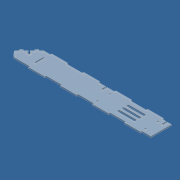
# Autodesk Inventor part: Wall
Saved by Autodesk Inventor 2016 (Build 200138000, 138)
## iProperties
Created: 2016-04-03
Part Number: Wall
Material: Polycarbonate, Clear
Document SubType Name: Modeling
Designer: admin
Density: 1.2 g/cm^3
Appearance: Polycarbonate - Clear
Author: admin
Autodesk Inventor part; units mm, degrees
ref_plane "YZ Plane" through (0, 0, 0) normal (1, 0, 0) x (0, 1, 0)
ref_plane "XZ Plane" through (0, 0, 0) normal (0, 1, 0) x (-1, 0, 0)
ref_plane "XY Plane" through (0, 0, 0) normal (0, 0, 1) x (1, 0, 0)
sketch "Sketch1" plane through (0, 0, 0) normal (0, 0, 1) x (1, 0, 0)
  line L0 (142.5, -22.5) -> (142.5, 22.5)
  arc A0 (-169.3198, -9.3198) -> (-157.5, -22.5) centre (-130.5627, 13.547) ccw
  line L1 (-154.4706, 5.5294) -> (-150.935, 1.9939)
  line L2 (-150.935, 1.9939) -> (-152.2157, 0.7132)
  line L3 (-152.2157, 0.7132) -> (-150.8015, -0.701)
  line L4 (-150.8015, -0.701) -> (-149.5208, 0.5797)
  line L5 (-149.5208, 0.5797) -> (-147.3995, -1.5416)
  line L6 (-147.3995, -1.5416) -> (-145.2782, 0.5797)
  line L7 (-145.2782, 0.5797) -> (-147.3995, 2.701)
  line L8 (-147.3995, 2.701) -> (-146.1188, 3.9817)
  line L9 (-146.1188, 3.9817) -> (-147.533, 5.3959)
  line L10 (-147.533, 5.3959) -> (-148.8137, 4.1152)
  line L11 (-148.8137, 4.1152) -> (-152.3492, 7.6508)
  line L12 (-154.542, 7.7222) -> (-156.666, 9.8462) construction
  line L13 (-122.5, 22.5) -> (-122.5, 25.5)
  line L14 (-122.5, 25.5) -> (-87.5, 25.5)
  line L15 (-87.5, 25.5) -> (-87.5, 22.5)
  line L16 (-52.5, 22.5) -> (-52.5, 25.5)
  line L17 (-52.5, 25.5) -> (-17.5, 25.5)
  line L18 (-17.5, 25.5) -> (-17.5, 22.5)
  line L19 (17.5, 22.5) -> (17.5, 25.5)
  line L20 (17.5, 25.5) -> (52.5, 25.5)
  line L21 (52.5, 25.5) -> (52.5, 22.5)
  line L22 (87.5, 22.5) -> (87.5, 25.5)
  line L23 (87.5, 25.5) -> (122.5, 25.5)
  line L24 (122.5, 25.5) -> (122.5, 22.5)
  line L25 (87.5, 22.5) -> (52.5, 22.5)
  line L26 (-52.5, 22.5) -> (-87.5, 22.5)
  line L27 (-122.5, 22.5) -> (-137.5, 22.5)
  line L28 (-122.5, -22.5) -> (-122.5, -25.5)
  line L29 (-122.5, -25.5) -> (-87.5, -25.5)
  line L30 (-87.5, -25.5) -> (-87.5, -22.5)
  line L31 (-52.5, -22.5) -> (-52.5, -25.5)
  line L32 (-52.5, -25.5) -> (-17.5, -25.5)
  line L33 (-17.5, -25.5) -> (-17.5, -22.5)
  line L34 (17.5, -22.5) -> (17.5, -25.5)
  line L35 (17.5, -25.5) -> (52.5, -25.5)
  line L36 (52.5, -25.5) -> (52.5, -22.5)
  line L37 (87.5, -22.5) -> (87.5, -25.5)
  line L38 (87.5, -25.5) -> (122.5, -25.5)
  line L39 (122.5, -25.5) -> (122.5, -22.5)
  line L40 (-157.5, -22.5) -> (-122.5, -22.5)
  line L41 (-87.5, -22.5) -> (-52.5, -22.5)
  line L42 (-17.5, -22.5) -> (17.5, -22.5)
  line L43 (52.5, -22.5) -> (87.5, -22.5)
  line L44 (122.5, -22.5) -> (142.5, -22.5)
  line L45 (-1.5, 12.5) -> (-1.5, 22.5)
  line L46 (1.5, 22.5) -> (1.5, 12.5)
  line L47 (1.5, 12.5) -> (-1.5, 12.5)
  line L48 (-37.337, 0) -> (-30.889, 0) construction
  line L49 (-164.0165, -4.0165) -> (-166.1378, -1.8952)
  line L50 (-166.1378, -1.8952) -> (-161.8952, 2.3475)
  line L51 (-161.8952, 2.3475) -> (-159.7739, 0.2261)
  line L52 (-147.0459, 12.9541) -> (-149.1673, 15.0754)
  line L53 (-149.1673, 15.0754) -> (-144.9246, 19.318)
  line L54 (-144.9246, 19.318) -> (-142.8033, 17.1967)
  line L55 (-154.4706, 5.5294) -> (-159.7739, 0.2261)
  line L56 (-164.0165, -4.0165) -> (-169.3198, -9.3198)
  line L57 (-137.5, 22.5) -> (-142.8033, 17.1967)
  line L58 (-147.0459, 12.9541) -> (-152.3492, 7.6508)
  line L59 (17.5, 22.5) -> (1.5, 22.5)
  line L60 (-1.5, 22.5) -> (-17.5, 22.5)
  line L61 (131, 22.5) -> (131, 12.5)
  line L62 (131, 12.5) -> (134, 12.5)
  line L63 (134, 12.5) -> (134, 22.5)
  line L64 (122.5, 22.5) -> (131, 22.5)
  line L65 (134, 22.5) -> (142.5, 22.5)
  point P0 (0, 0)
  point P1 (142.5, 0)
  point P2 (-146.3388, -0.481)
  point P3 (0, -22.5)
  point P4 (1.5, -22.5)
  dimension "d0" = 45
  dimension "d2" = 45
  dimension "d4" = 45
  dimension "d7" = 3
  dimension "d8" = 2
  dimension "d9" = 3
  dimension "d10" = 5
  dimension "d11" = 6.6223
  dimension "d13" = 35
  dimension "d15" = 20
  dimension "d17" = 10
  dimension "d23" = 45
  dimension "d24" = 6
  dimension "d25" = 18
  dimension "d35" = 3
  dimension "d36" = 35
  dimension "d37" = 15
  dimension "d38" = 300
  dimension "d40" = 8.5
  constraints: 132 end point, 72 perpendicular, 33 collinear, 16 equal length, 8 horizontal, 6 parallel, 5 vertical, 3 midpoint, 2 point on circle, 2 point on line, 1 centre point, 1 horizontal alignment, 1 vertical alignment, 2 other
  measures "d0" distance of L0.start L0.end
  measures "d2" distance of L56.end L27.end
  measures "d4" radius of A0
  measures "d7" distance between parallel lines of L7 L5
  measures "d8" distance between parallel lines of L8 L10
  measures "d9" distance of L6.end L7.end
  measures "d10" distance of L10.end L11.end
  measures "d11" distance between parallel lines of L9 L3
  measures "d13" distance of L13.end L14.end
  measures "d15" distance from line of L23.end L0
  measures "d17" distance of L45.start L45.end
  measures "d23" angle of L40 L56
  measures "d24" distance of L49.end L50.end
  measures "d25" distance between parallel lines of L52 L51
  measures "d35" distance of L22.start L22.end
  measures "d36" distance of L19.start L18.end
  measures "d37" distance of L13.start L27.end
  measures "d38" distance from line of L0 L40.start
  measures "d40" distance between parallel lines of L0 L63
extrude "Extrusion1" add sketch "Sketch1" along normal blind 3
sketch "Sketch2" plane through (0, 0, 3) normal (0, 0, 1) x (1, 0, 0)
  line L0 (1.5, 22.5) -> (1.5, 12.5) projected
  line L1 (142.5, -22.5) -> (142.5, 22.5) projected
  line L2 (122.5, 22.5) -> (122.5, 25.5) projected
  line L3 (122.5, 25.5) -> (87.5, 25.5) projected
  line L4 (87.5, 25.5) -> (87.5, 22.5) projected
  line L5 (87.5, 22.5) -> (52.5, 22.5) projected
  line L6 (52.5, 22.5) -> (52.5, 25.5) projected
  line L7 (52.5, 25.5) -> (17.5, 25.5) projected
  line L8 (17.5, 25.5) -> (17.5, 22.5) projected
  line L9 (17.5, 22.5) -> (1.5, 22.5) projected
  line L10 (-17.5, -22.5) -> (17.5, -22.5) projected
  line L11 (17.5, -22.5) -> (17.5, -25.5) projected
  line L12 (17.5, -25.5) -> (52.5, -25.5) projected
  line L13 (52.5, -25.5) -> (52.5, -22.5) projected
  line L14 (52.5, -22.5) -> (87.5, -22.5) projected
  line L15 (87.5, -22.5) -> (87.5, -25.5) projected
  line L16 (87.5, -25.5) -> (122.5, -25.5) projected
  line L17 (122.5, -25.5) -> (122.5, -22.5) projected
  line L18 (122.5, -22.5) -> (142.5, -22.5) projected
  line L19 (-125.5, 10) -> (-125.5, -10)
  line L20 (131, 22.5) -> (122.5, 22.5) projected
  line L21 (1.5, 12.5) -> (-1.5, 12.5) projected
  line L22 (-1.5, 12.5) -> (-1.5, 22.5) projected
  line L23 (-1.5, 22.5) -> (-17.5, 22.5) projected
  line L24 (-17.5, 22.5) -> (-17.5, 25.5) projected
  line L25 (-17.5, 25.5) -> (-52.5, 25.5) projected
  line L26 (-52.5, 25.5) -> (-52.5, 22.5) projected
  line L27 (-52.5, 22.5) -> (-87.5, 22.5) projected
  line L28 (-87.5, 22.5) -> (-87.5, 25.5) projected
  line L29 (-87.5, 25.5) -> (-122.5, 25.5) projected
  line L30 (-122.5, 25.5) -> (-122.5, 22.5) projected
  line L31 (-122.5, -25.5) -> (-87.5, -25.5) projected
  line L32 (-87.5, -25.5) -> (-87.5, -22.5) projected
  line L33 (-87.5, -22.5) -> (-52.5, -22.5) projected
  line L34 (-52.5, -22.5) -> (-52.5, -25.5) projected
  line L35 (-52.5, -25.5) -> (-17.5, -25.5) projected
  line L36 (-17.5, -25.5) -> (-17.5, -22.5) projected
  line L37 (-122.5, 22.5) -> (-137.5, 22.5) projected
  line L38 (-137.5, 22.5) -> (-142.8033, 17.1967) projected
  line L39 (-142.8033, 17.1967) -> (-144.9246, 19.318) projected
  line L40 (-144.9246, 19.318) -> (-149.1673, 15.0754) projected
  line L41 (-149.1673, 15.0754) -> (-147.0459, 12.9541) projected
  line L42 (-147.0459, 12.9541) -> (-152.3492, 7.6508) projected
  line L43 (-152.3492, 7.6508) -> (-148.8137, 4.1152) projected
  line L44 (-148.8137, 4.1152) -> (-147.533, 5.3959) projected
  line L45 (-147.533, 5.3959) -> (-146.1188, 3.9817) projected
  line L46 (-146.1188, 3.9817) -> (-147.3995, 2.701) projected
  line L47 (-147.3995, 2.701) -> (-145.2782, 0.5797) projected
  line L48 (-157.5, -22.5) -> (-122.5, -22.5) projected
  line L49 (-122.5, -22.5) -> (-122.5, -25.5) projected
  line L50 (-145.2782, 0.5797) -> (-147.3995, -1.5416) projected
  line L51 (-147.3995, -1.5416) -> (-149.5208, 0.5797) projected
  line L52 (-149.5208, 0.5797) -> (-150.8015, -0.701) projected
  line L53 (-150.8015, -0.701) -> (-152.2157, 0.7132) projected
  line L54 (-152.2157, 0.7132) -> (-150.935, 1.9939) projected
  line L55 (-150.935, 1.9939) -> (-154.4706, 5.5294) projected
  line L56 (-154.4706, 5.5294) -> (-159.7739, 0.2261) projected
  line L57 (-159.7739, 0.2261) -> (-161.8952, 2.3475) projected
  line L58 (-161.8952, 2.3475) -> (-166.1378, -1.8952) projected
  line L59 (-166.1378, -1.8952) -> (-164.0165, -4.0165) projected
  line L60 (-164.0165, -4.0165) -> (-169.3198, -9.3198) projected
  arc A0 (-169.3198, -9.3198) -> (-157.5, -22.5) centre (-130.5627, 13.547) ccw projected
  line L61 (142.5, 22.5) -> (134, 22.5) projected
  line L62 (134, 22.5) -> (134, 12.5) projected
  line L63 (134, 12.5) -> (131, 12.5) projected
  line L64 (131, 12.5) -> (131, 22.5) projected
  line L65 (-125.5, 10) -> (-122.5, 10)
  line L66 (-122.5, 10) -> (-122.5, -10)
  line L67 (-122.5, -10) -> (-125.5, -10)
  line L68 (-87.5, 22.5) -> (-87.5, 25.5) projected
  point P0 (0, 0)
  point P1 (-125.5, 0)
  dimension "d20" = 268
  dimension "d39" = 20
  constraints: 8 end point, 2 horizontal, 1 horizontal alignment, 1 midpoint, 1 perpendicular, 1 vertical
  measures "d20" distance between parallel lines of L1 L19
  measures "d39" distance between parallel lines of L67 L65
extrude "Extrusion2" cut sketch "Sketch2" against normal blind 10 contours L65 L66 L67 L19
sketch "Sketch3" plane through (0, 0, 3) normal (0, 0, 1) x (1, 0, 0)
  line L0 (1.5, 22.5) -> (1.5, 12.5) projected
  line L1 (142.5, -22.5) -> (142.5, 22.5) projected
  line L2 (122.5, 22.5) -> (122.5, 25.5) projected
  line L3 (122.5, 25.5) -> (87.5, 25.5) projected
  line L4 (87.5, 25.5) -> (87.5, 22.5) projected
  line L5 (87.5, 22.5) -> (52.5, 22.5) projected
  line L6 (52.5, 22.5) -> (52.5, 25.5) projected
  line L7 (52.5, 25.5) -> (17.5, 25.5) projected
  line L8 (17.5, 25.5) -> (17.5, 22.5) projected
  line L9 (17.5, 22.5) -> (1.5, 22.5) projected
  line L10 (-17.5, -22.5) -> (17.5, -22.5) projected
  line L11 (17.5, -22.5) -> (17.5, -25.5) projected
  line L12 (17.5, -25.5) -> (52.5, -25.5) projected
  line L13 (52.5, -25.5) -> (52.5, -22.5) projected
  line L14 (52.5, -22.5) -> (87.5, -22.5) projected
  line L15 (87.5, -22.5) -> (87.5, -25.5) projected
  line L16 (87.5, -25.5) -> (122.5, -25.5) projected
  line L17 (122.5, -25.5) -> (122.5, -22.5) projected
  line L18 (122.5, -22.5) -> (142.5, -22.5) projected
  arc A0 (59.5166, -6.8198) -> (59.5166, -11.8198) centre (59.5166, -9.3198) ccw
  arc A1 (94.5166, -11.8198) -> (94.5166, -6.8198) centre (94.5166, -9.3198) ccw
  line L19 (59.5166, -6.8198) -> (94.5166, -6.8198)
  line L20 (59.5166, -11.8198) -> (94.5166, -11.8198)
  line L21 (131, 22.5) -> (122.5, 22.5) projected
  line L22 (1.5, 12.5) -> (-1.5, 12.5) projected
  line L23 (-1.5, 12.5) -> (-1.5, 22.5) projected
  line L24 (-1.5, 22.5) -> (-17.5, 22.5) projected
  line L25 (-17.5, 22.5) -> (-17.5, 25.5) projected
  line L26 (-17.5, 25.5) -> (-52.5, 25.5) projected
  line L27 (-52.5, 25.5) -> (-52.5, 22.5) projected
  line L28 (-52.5, 22.5) -> (-87.5, 22.5) projected
  line L29 (-87.5, 22.5) -> (-87.5, 25.5) projected
  line L30 (-87.5, 25.5) -> (-122.5, 25.5) projected
  line L31 (-122.5, -22.5) -> (-122.5, -25.5) projected
  line L32 (-122.5, -25.5) -> (-87.5, -25.5) projected
  line L33 (-87.5, -25.5) -> (-87.5, -22.5) projected
  line L34 (-87.5, -22.5) -> (-52.5, -22.5) projected
  line L35 (-52.5, -22.5) -> (-52.5, -25.5) projected
  line L36 (-52.5, -25.5) -> (-17.5, -25.5) projected
  line L37 (-17.5, -25.5) -> (-17.5, -22.5) projected
  line L38 (-122.5, 22.5) -> (-137.5, 22.5) projected
  line L39 (-137.5, 22.5) -> (-142.8033, 17.1967) projected
  line L40 (-142.8033, 17.1967) -> (-144.9246, 19.318) projected
  line L41 (-144.9246, 19.318) -> (-149.1673, 15.0754) projected
  line L42 (-149.1673, 15.0754) -> (-147.0459, 12.9541) projected
  line L43 (-147.0459, 12.9541) -> (-152.3492, 7.6508) projected
  line L44 (-157.5, -22.5) -> (-122.5, -22.5) projected
  line L45 (-164.0165, -4.0165) -> (-169.3198, -9.3198) projected
  arc A2 (-169.3198, -9.3198) -> (-157.5, -22.5) centre (-130.5627, 13.547) ccw projected
  line L46 (-125.5, -10) -> (-125.5, 10) projected
  line L47 (142.5, 22.5) -> (134, 22.5) projected
  line L48 (134, 22.5) -> (134, 12.5) projected
  line L49 (134, 12.5) -> (131, 12.5) projected
  line L50 (131, 12.5) -> (131, 22.5) projected
  line L51 (-122.5, -10) -> (-125.5, -10) projected
  line L52 (-125.5, 10) -> (-122.5, 10) projected
  line L53 (-122.5, 10) -> (-122.5, -10) projected
  line L54 (-152.3492, 7.6508) -> (-148.8137, 4.1152) projected
  line L55 (-148.8137, 4.1152) -> (-147.533, 5.3959) projected
  line L56 (-147.533, 5.3959) -> (-146.1188, 3.9817) projected
  line L57 (-146.1188, 3.9817) -> (-147.3995, 2.701) projected
  line L58 (-147.3995, 2.701) -> (-145.2782, 0.5797) projected
  line L59 (-145.2782, 0.5797) -> (-147.3995, -1.5416) projected
  line L60 (-147.3995, -1.5416) -> (-149.5208, 0.5797) projected
  line L61 (-149.5208, 0.5797) -> (-150.8015, -0.701) projected
  line L62 (-150.8015, -0.701) -> (-152.2157, 0.7132) projected
  line L63 (-152.2157, 0.7132) -> (-150.935, 1.9939) projected
  line L64 (-150.935, 1.9939) -> (-154.4706, 5.5294) projected
  line L65 (-154.4706, 5.5294) -> (-159.7739, 0.2261) projected
  line L66 (-159.7739, 0.2261) -> (-161.8952, 2.3475) projected
  line L67 (-161.8952, 2.3475) -> (-166.1378, -1.8952) projected
  line L68 (-166.1378, -1.8952) -> (-164.0165, -4.0165) projected
  line L69 (-122.5, 25.5) -> (-122.5, 22.5) projected
  point P0 (0, 0)
  dimension "d26" = 5
  dimension "d27" = 35
  constraints: 4 end point, 4 point on circle, 3 tangent, 2 centre point, 1 equal radius, 1 horizontal, 1 horizontal alignment
  measures "d26" diameter of A0
  measures "d27" distance of A1.centre A0.centre
extrude "Extrusion3" cut sketch "Sketch3" against normal up to next contours L19 A1 L20 A0
pattern_linear "Rectangular Pattern1" count 3 spacing 10 along (0, 1, 0) of "Extrusion3"
sketch "Sketch4" plane through (0, 0, 3) normal (0, 0, 1) x (1, 0, 0)
  line L0 (1.5, 22.5) -> (1.5, 12.5) projected
  line L1 (-17.4416, 0) -> (12.3581, 0) construction
  point P0 (0, 0)
  point P1 (16.5, 13.5)
  point P2 (16.5, -13.5)
  point P3 (121.5, 13.5)
  point P4 (121.5, -13.5)
  dimension "d41" = 27
  dimension "d42" = 15
  dimension "d43" = 105
  constraints: 2 end point, 2 horizontal alignment, 2 vertical alignment, 1 horizontal, 1 point on line, 1 symmetric about line
  measures "d41" distance of point (16.5, -13.5) point (16.5, 13.5)
  measures "d42" distance from line of point (16.5, 13.5) L0
  measures "d43" distance of point (16.5, 13.5) point (121.5, 13.5)
hole "Hole1" at (16.5, 13.5, 3) at (16.5, -13.5, 3) at (121.5, 13.5, 3) at (121.5, -13.5, 3) direction (0, 0, -1) diameter 3 end through all countersink diameter 5 countersink angle 90
body "Solid1"
